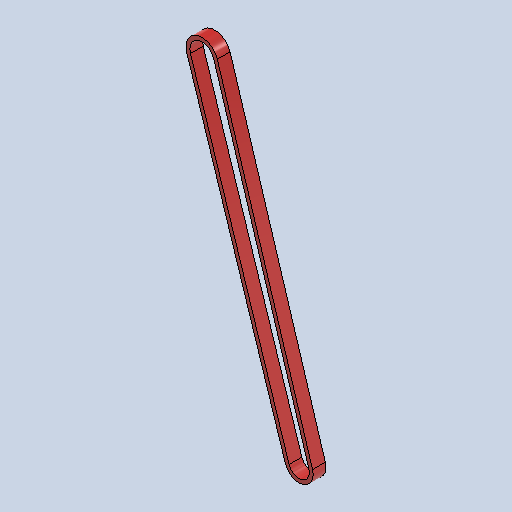
# Autodesk Inventor part: Angle Changer right band
Saved by Autodesk Inventor 2023.2 (Build 272271030, 271C)
## iProperties
Created: 2023-04-07
Part Number: Angle Changer right band
Material: Generic
Document SubType Name: Modeling
Designer: Main Account
Density: 1 g/cm^3
Appearance: Default
Author: Main Account
Autodesk Inventor part; units mm, degrees
ref_plane "YZ Plane" through (0, 0, 0) normal (1, 0, 0) x (0, 1, 0)
ref_plane "XZ Plane" through (0, 0, 0) normal (0, 1, 0) x (-1, 0, 0)
ref_plane "XY Plane" through (0, 0, 0) normal (0, 0, 1) x (1, 0, 0)
sketch "Sketch1" plane through (0, 0, 0) normal (0, 0, 1) x (1, 0, 0)
  circle A0 centre (0, 0) radius 4.7625 construction
  circle A1 centre (37.9719, -120.3156) radius 2.1844 construction
  arc A2 (34.1032, -121.5602) -> (41.8542, -119.1139) centre (37.9719, -120.3156) ccw
  arc A3 (4.5495, 1.4082) -> (-4.5337, -1.4585) centre (0, 0) ccw
  line L0 (-4.5337, -1.4585) -> (34.1032, -121.5602)
  line L1 (41.8542, -119.1139) -> (4.5495, 1.4082)
  line L2 (32.6752, -122.0195) -> (-5.9616, -1.9179)
  arc A4 (5.9825, 1.8517) -> (-5.9616, -1.9179) centre (0, 0) ccw
  line L3 (5.9825, 1.8517) -> (43.2871, -118.6704)
  arc A5 (32.6752, -122.0195) -> (43.2871, -118.6704) centre (37.9719, -120.3156) ccw
  point P0 (0, 0)
  dimension "d0" = 8.128
  dimension "d1" = 1.5
  constraints: 8 end point, 8 point on circle, 4 centre point, 4 tangent, 2 coincident, 1 concentric, 3 other
  measures "d0" diameter of A2
  measures "d1" distance between parallel lines of L0 L2
extrude "Extrusion1" add sketch "Sketch1" along normal blind 5
body "Solid1"
